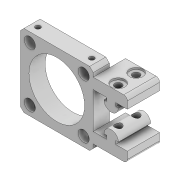
# Autodesk Inventor part: Rain_LensHolder
Saved by Autodesk Inventor 2022 (Build 260153000, 153)
## iProperties
Created: 2022-06-21
Part Number: Rain_LensHolder
Material: Generic
Document SubType Name: Modeling
Designer: wanghaoran
Density: 1 g/cm^3
Appearance: Default
Author: wanghaoran
Autodesk Inventor part; units mm, degrees
ref_plane "YZ Plane" through (0, 0, 0) normal (1, 0, 0) x (0, 1, 0)
ref_plane "XZ Plane" through (0, 0, 0) normal (0, 1, 0) x (-1, 0, 0)
ref_plane "XY Plane" through (0, 0, 0) normal (0, 0, 1) x (1, 0, 0)
sketch "Sketch1" plane through (0, 0, 0) normal (0, 0, 1) x (1, 0, 0)
  line L0 (-20, -85.8136) -> (-20, -78.3136) projected
  line L1 (-20, -78.3136) -> (-18.5, -78.3136) projected
  line L2 (-18.5, -78.3136) -> (-18.5, -82.5636) projected
  line L3 (-18.5, -82.5636) -> (-17.8462, -82.5636) projected
  line L4 (-17.8462, -82.5636) -> (-14, -78.7175) projected
  line L5 (-14, -78.7175) -> (-14, -72.9098) projected
  line L6 (-14, -72.9098) -> (-17.8462, -69.0636) projected
  line L7 (-17.8462, -69.0636) -> (-18.5, -69.0636) projected
  line L8 (-18.5, -69.0636) -> (-18.5, -73.3136) projected
  line L9 (-18.5, -73.3136) -> (-20, -73.3136) projected
  line L10 (-20, -73.3136) -> (-20, -65.8136) projected
  line L11 (-20, -65.8136) -> (-12.5, -65.8136) projected
  line L12 (-12.5, -65.8136) -> (-12.5, -67.3136) projected
  line L13 (-12.5, -67.3136) -> (-16.75, -67.3136) projected
  line L14 (-16.75, -67.3136) -> (-16.75, -68.0385) projected
  line L15 (-16.75, -68.0385) -> (-12.9748, -71.8136) projected
  line L16 (-12.9748, -71.8136) -> (-7.0252, -71.8136) projected
  line L17 (-7.0252, -71.8136) -> (-3.25, -68.0385) projected
  line L18 (-3.25, -68.0385) -> (-3.25, -67.3136) projected
  line L19 (-3.25, -67.3136) -> (-7.5, -67.3136) projected
  line L20 (-7.5, -67.3136) -> (-7.5, -65.8136) projected
  line L21 (-7.5, -65.8136) -> (0, -65.8136) projected
  line L22 (0, -65.8136) -> (0, -73.3136) projected
  line L23 (0, -73.3136) -> (-1.5, -73.3136) projected
  line L24 (-1.5, -73.3136) -> (-1.5, -69.0636) projected
  line L25 (-1.5, -69.0636) -> (-2.1538, -69.0636) projected
  line L26 (-2.1538, -69.0636) -> (-6, -72.9098) projected
  line L27 (-6, -72.9098) -> (-6, -78.7175) projected
  line L28 (-6, -78.7175) -> (-2.1538, -82.5636) projected
  line L29 (-2.1538, -82.5636) -> (-1.5, -82.5636) projected
  line L30 (-1.5, -82.5636) -> (-1.5, -78.3136) projected
  line L31 (-1.5, -78.3136) -> (0, -78.3136) projected
  line L32 (0, -78.3136) -> (0, -85.8136) projected
  line L33 (0, -85.8136) -> (-7.5, -85.8136) projected
  line L34 (-7.5, -85.8136) -> (-7.5, -84.3136) projected
  line L35 (-7.5, -84.3136) -> (-3.25, -84.3136) projected
  line L36 (-3.25, -84.3136) -> (-3.25, -83.5888) projected
  line L37 (-3.25, -83.5888) -> (-7.0252, -79.8136) projected
  line L38 (-7.0252, -79.8136) -> (-12.9748, -79.8136) projected
  line L39 (-12.9748, -79.8136) -> (-16.75, -83.5888) projected
  line L40 (-16.75, -83.5888) -> (-16.75, -84.3136) projected
  line L41 (-16.75, -84.3136) -> (-12.5, -84.3136) projected
  line L42 (-12.5, -84.3136) -> (-12.5, -85.8136) projected
  line L43 (-12.5, -85.8136) -> (-20, -85.8136) projected
  circle A0 centre (-10, -75.8136) radius 2.15 projected
  line L44 (-12.5, -65.7136) -> (-7.5, -65.7136)
  line L45 (-7.5, -65.7136) -> (-7.5, -67.6136)
  line L46 (-7.5, -67.6136) -> (-12.5, -67.6136)
  line L47 (-12.5, -67.6136) -> (-12.5, -65.7136)
  line L48 (-12.5, -67.6136) -> (-14, -67.6136)
  line L49 (-7.5, -67.6136) -> (-6, -67.6136)
  arc A1 (-14, -67.6136) -> (-6, -67.6136) centre (-10, -67.6136) ccw
  line L50 (-20, -65.8136) -> (-20, -59.8136)
  line L51 (-14, -75.8136) -> (-32.3565, -75.8136)
  line L52 (-20, -75.8136) -> (-60.6, -75.8136)
  line L53 (-60.6, -75.8136) -> (-60.6, -57.5136)
  line L54 (-58.6, -55.5136) -> (-22, -55.5136)
  line L55 (-20, -57.5136) -> (-20, -75.8136)
  line L56 (-22, -55.5136) -> (-20, -57.5136)
  line L57 (-60.6, -57.5136) -> (-58.6, -55.5136)
  arc A2 (-24.8, -75.8136) -> (-55.8, -75.8136) centre (-40.3, -75.8136) ccw
  circle A3 centre (-55.3, -60.8136) radius 3.1
  circle A4 centre (-25.3, -60.8136) radius 3.1
  line L58 (-20, -65.7136) -> (-1, -65.7136)
  line L59 (-1, -65.7136) -> (-1, -61.7136)
  line L60 (-3, -59.7136) -> (-20, -59.7136)
  line L61 (-20, -59.7136) -> (-20, -65.7136)
  arc A5 (-1, -61.7136) -> (-3, -59.7136) centre (-3, -61.7136) ccw
  point P0 (0, 0)
  point P1 (-1, -65.8136)
  point P2 (-1, -59.8136)
  point P3 (-60.6, -55.5136)
  point P4 (-20, -55.5136)
  point P5 (-1, -59.7136)
  point P6 (-20, -65.7136)
  point P7 (-12.5, -65.7136)
  point P8 (-7.5, -65.7136)
  dimension "d3" = 5
  dimension "d4" = 1.9
  dimension "d6" = 0
  dimension "d7" = 1.5
  dimension "d8" = 1.5
  dimension "d9" = 4
  dimension "d10" = 19
  dimension "d11" = 6
  dimension "d15" = 40.6
  dimension "d16" = 20.3
  dimension "d17" = 2
  dimension "d18" = 2
  dimension "d19" = 2
  dimension "d20" = 2
  dimension "d21" = 31
  dimension "d22" = 6.2
  dimension "d23" = 5.3
  dimension "d24" = 5.3
  dimension "d25" = 6.2
  dimension "d26" = 5.3
  dimension "d27" = 5.3
  dimension "d32" = 0.3
  dimension "d33" = 19
  dimension "d34" = 6
  dimension "d35" = 2
  dimension "d58" = 4.2
  constraints: 36 end point, 11 point on line, 6 parallel, 6 point on circle, 5 centre point, 5 horizontal, 3 perpendicular, 2 midpoint, 2 tangent
  measures "d3" distance of L45.end L46.end
  measures "d4" distance of L46.end L44.start
  measures "d6" distance between parallel lines of L12 L47
  measures "d7" distance of L46.end L48.end
  measures "d8" distance of L45.end L49.end
  measures "d9" radius of A1
  measures "d10" distance of L50.end point (-1, -59.814)
  measures "d11" distance of L50.start L50.end
  measures "d15" distance of point (-60.6, -55.514) point (-20, -55.514)
  measures "d16" distance of L52.end point (-60.6, -55.514)
  measures "d17" distance of L54.end point (-20, -55.514)
  measures "d18" distance of L55.start point (-20, -55.514)
  measures "d19" distance of L53.end point (-60.6, -55.514)
  measures "d20" distance of L54.start point (-60.6, -55.514)
  measures "d21" diameter of A2
  measures "d22" diameter of A3
  measures "d23" distance from line of L53 A3.centre
  measures "d24" distance from line of L54 A3.centre
  measures "d25" diameter of A4
  measures "d26" distance from line of L10 A4.centre
  measures "d27" distance from line of L54 A4.centre
  measures "d32" distance between parallel lines of L13 L48
  measures "d33" distance of L60.end point (-1, -59.714)
  measures "d34" distance of point (-1, -59.714) L58.end
  measures "d35" radius of A5
  measures "d58" distance between parallel lines of L54 L60
extrude "Extrusion1" add sketch "Sketch1" along normal blind 9 contours L51 A2 L52 L53 L57 L54 L56 L55 L50 L10 | L47 L44 L45 L20 L46 L12 | L50 L55 L60 A5 L59 L58 L44 | L46 L49 A1 L48
sketch "Sketch4" plane through (0, 0, 0) normal (0, 0, -1) x (-1, 0, 0)
  line L0 (22, -55.5136) -> (58.6, -55.5136) projected
  line L1 (20, -57.5136) -> (22, -55.5136) projected
  line L2 (20, -59.7136) -> (20, -57.5136) projected
  line L3 (3, -59.7136) -> (20, -59.7136) projected
  arc A0 (3, -59.7136) -> (1, -61.7136) centre (3, -61.7136) ccw projected
  line L4 (1, -65.7136) -> (1, -61.7136) projected
  line L5 (7.5, -65.7136) -> (1, -65.7136) projected
  line L6 (7.5, -67.6136) -> (7.5, -65.7136) projected
  line L7 (6, -67.6136) -> (7.5, -67.6136) projected
  arc A1 (6, -67.6136) -> (14, -67.6136) centre (10, -67.6136) ccw projected
  line L8 (12.5, -67.6136) -> (14, -67.6136) projected
  line L9 (12.5, -65.7136) -> (12.5, -67.6136) projected
  line L10 (20, -65.7136) -> (12.5, -65.7136) projected
  line L11 (20, -75.8136) -> (20, -65.7136) projected
  line L12 (24.8, -75.8136) -> (20, -75.8136) projected
  arc A2 (55.8, -75.8136) -> (24.8, -75.8136) centre (40.3, -75.8136) ccw projected
  line L13 (60.6, -75.8136) -> (55.8, -75.8136) projected
  line L14 (60.6, -57.5136) -> (60.6, -75.8136) projected
  line L15 (58.6, -55.5136) -> (60.6, -57.5136) projected
  circle A3 centre (25.3, -60.8136) radius 3.1 projected
  circle A4 centre (55.3, -60.8136) radius 3.1 projected
  line L16 (20, -59.7136) -> (20, -57.5136) projected
  line L17 (20, -75.8136) -> (20, -65.7136) projected
  line L18 (20, -59.7136) -> (20, -65.7136)
  point P0 (0, 0)
  constraints: 2 end point, 1 vertical
extrude "Extrusion3" add sketch "Sketch4" along normal blind 9 contours L18 L10 L9 L8 A1 L7 L6 L5 L4 A0 L3
sketch "Sketch5" plane through (-20, -59.7136, 9) normal (0, 1, 0) x (1, 0, 0)
  line L0 (6, 18) -> (6, 0) projected
  line L1 (14, 18) -> (14, 0) projected
  circle A0 centre (9.9, 4) radius 1.95
  circle A1 centre (9.9, 14) radius 1.95
  line L2 (0, 18) -> (17, 18) projected
  line L3 (17, 0) -> (0, 0) projected
  point P0 (20, 9)
  dimension "d38" = 3.9
  dimension "d39" = 3.9
  dimension "d40" = 3.9
  dimension "d41" = 3.9
  dimension "d42" = 4
  dimension "d43" = 4
  constraints: 2 centre point
  measures "d38" diameter of A0
  measures "d39" diameter of A1
  measures "d40" distance from line of L0 A0.centre
  measures "d41" distance from line of L0 A1.centre
  measures "d42" distance from line of L2 A1.centre
  measures "d43" distance from line of L3 A0.centre
hole "Hole1" at (-10.1, -59.7136, 5) at (-10.1, -59.7136, -5) direction (0, -1, 0) diameter 3.9 end through all counterbore diameter 7.4 counterbore depth 1
sketch "Sketch6" plane through (0, -55.5136, 0) normal (0, 1, 0) x (-1, 0, 0)
  line L0 (52.2, 9) -> (58.4, 9) projected
  line L1 (52.2, 0) -> (58.4, 0) projected
  line L2 (22.2, 9) -> (28.4, 9) projected
  line L3 (22.2, 0) -> (28.4, 0) projected
  circle A0 centre (55.3, 4.5) radius 1.4
  circle A1 centre (25.3, 4.5) radius 1.4
  line L4 (52.2, 9) -> (58.4, 9) projected
  line L5 (58.6, 0) -> (58.6, 9)
  line L6 (58.4, 9) -> (58.4, 0)
  line L7 (22, 9) -> (58.6, 9) projected
  point P0 (0, 0)
  dimension "d51" = 2.8
  dimension "d52" = 2.8
  dimension "d53" = 4.5
  dimension "d54" = 4.5
  constraints: 4 end point, 2 centre point, 1 perpendicular
  measures "d51" diameter of A0
  measures "d52" diameter of A1
  measures "d53" distance from line of L1 A0.centre
  measures "d54" distance from line of L3 A1.centre
extrude "Extrusion4" cut sketch "Sketch6" against normal blind 4
mirror "Mirror1" about plane through (-60.6, -75.8136, 0) normal (0, -1, 0) of "Extrusion1", "Extrusion3", "Hole1", "Extrusion4"
equation "\"d18\" = d17"
equation "\"d19\" = d17"
equation "\"d20\" = d19"
body "Solid1"
